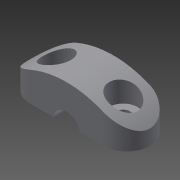
# Autodesk Inventor part: YAxisRodClamp
Saved by Autodesk Inventor 2015 (Build 190159000, 159)
## iProperties
Created: 2014-08-08
Part Number: YAxisRodClamp
Material: Generic
Document SubType Name: Modeling
Designer: t_clevj
Density: 1 g/cm^3
Appearance: Default
Author: t_clevj
Autodesk Inventor part; units mm, degrees
ref_plane "YZ Plane" through (0, 0, 0) normal (1, 0, 0) x (0, 1, 0)
ref_plane "XZ Plane" through (0, 0, 0) normal (0, 1, 0) x (-1, 0, 0)
ref_plane "XY Plane" through (0, 0, 0) normal (0, 0, 1) x (1, 0, 0)
sketch "Sketch1" plane through (0, 0, 0) normal (0, 1, 0) x (-1, 0, 0)
  line L0 (0, 0) -> (0, 4.5)
  line L1 (36, 0) -> (36, 4.5)
  arc A0 (36, 4.5) -> (0, 4.5) centre (18, -16.9476) ccw
  circle A1 centre (18, -0.6) radius 4
  line L2 (0, 0) -> (14.0453, 0)
  line L3 (36, 0) -> (21.9547, 0)
  dimension "d0" = 4.5
  dimension "d1" = 4.5
  dimension "d2" = 36
  dimension "d3" = 28
  dimension "d4" = 8
  dimension "d5" = 0.6
  dimension "d6" = 18
  constraints: 8 end point, 4 point on circle, 2 centre point, 2 vertical, 1 collinear, 1 horizontal, 1 point on line
  measures "d0" distance of L0.start L0.end
  measures "d1" distance of L1.start L1.end
  measures "d2" distance between parallel lines of L0 L1
  measures "d3" radius of A0
  measures "d4" diameter of A1
  measures "d5" vertical distance of L0.start A1.centre
  measures "d6" horizontal distance of L1.start A1.centre
extrude "Extrusion1" add sketch "Sketch1" along normal blind 14 contours L0 A0 L1 L3 A1 L2
fillet "Fillet1" radius 7 4 edges at (0, 14, 2.25) (0, 0, 2.25) (-36, 14, 2.25) (-36, 0, 2.25)
sketch "Sketch2" plane through (-14.0453, 0, 0) normal (0, 0, -1) x (-1, 0, 0)
  arc A0 (-7.0453, 14) -> (-7.0453, 0) centre (-7.0453, 7) ccw projected
  arc A1 (14.9547, 0) -> (14.9547, 14) centre (14.9547, 7) ccw projected
  line L0 (7.9095, 14) -> (14.9547, 14) projected
  line L1 (7.9095, 0) -> (7.9095, 14) projected
  line L2 (7.9095, 0) -> (14.9547, 0) projected
  circle A2 centre (-6.0453, 7) radius 2
  circle A3 centre (13.9547, 7) radius 2
  point P0 (-14.0453, 0)
  dimension "d19" = 4
  dimension "d20" = 4
  dimension "d22" = 20
  dimension "d23" = 1
  constraints: 2 centre point, 2 horizontal alignment
  measures "d19" diameter of A2
  measures "d20" diameter of A3
  measures "d22" distance of A3.centre A2.centre
  measures "d23" distance of A3.centre A1.centre
extrude "Extrusion2" cut sketch "Sketch2" against normal up to next contours A2 | A3
ref_plane "Work Plane1" through (-14.0453, 0, 4) normal (0, 0, -1) x (-1, 0, 0)
ref_plane "Work Plane2" through (-14.0453, 0, 4) normal (0, 0, -1) x (-1, 0, 0)
sketch "Sketch4" plane through (-14.0453, 0, 4) normal (0, 0, -1) x (-1, 0, 0)
  spline S0 degree 8 poles (-4.0453, 7) (-4.0453, 7.2106) (-4.0706, 7.4217) (-4.1215, 7.6308) (-4.1983, 7.8352) (-4.3013, 8.0322) (-4.4309, 8.2183) (-4.5873, 8.3896) (-4.9297, 8.6728) (-5.1107, 8.7908) (-5.3107, 8.8886) (-5.5255, 8.9613) (-5.7497, 9.0058) (-5.9775, 9.0205) (-6.2028, 9.006) (-6.6538, 8.92) (-6.8753, 8.8448) (-7.0808, 8.7428) (-7.2677, 8.6177) (-7.4339, 8.4735) (-7.5781, 8.3138) (-7.6994, 8.1426) (-7.9062, 7.7665) (-7.9875, 7.5586) (-8.0417, 7.3434) (-8.0687, 7.124) (-8.0685, 6.9033) (-8.0411, 6.6843) (-7.9865, 6.47) (-7.8339, 6.0848) (-7.7425, 5.9113) (-7.6304, 5.7458) (-7.498, 5.5912) (-7.3457, 5.4501) (-7.1746, 5.3258) (-6.9859, 5.2214) (-6.584, 5.0623) (-6.3712, 5.0057) (-6.148, 4.9757) (-5.9201, 4.9747) (-5.6938, 5.0036) (-5.4751, 5.0611) (-5.2697, 5.1441) (-4.8226, 5.3899) (-4.5988, 5.5699) (-4.4125, 5.7777) (-4.2643, 6.0055) (-4.1541, 6.2469) (-4.0813, 6.4964) (-4.0453, 6.7489) (-4.0453, 7) knots 0 0 0 0 0 0 0 0 0 0.147327 0.147327 0.147327 0.147327 0.147327 0.147327 0.147327 0.27552 0.27552 0.27552 0.27552 0.27552 0.27552 0.27552 0.413502 0.413502 0.413502 0.413502 0.413502 0.413502 0.413502 0.565351 0.565351 0.565351 0.565351 0.565351 0.565351 0.565351 0.6971 0.6971 0.6971 0.6971 0.6971 0.6971 0.6971 0.824412 0.824412 0.824412 0.824412 0.824412 0.824412 0.824412 1 1 1 1 1 1 1 1 1 projected
  circle A0 centre (-6.0453, 7) radius 2 projected
  spline S1 degree 8 poles (15.9547, 7) (15.9547, 7.1989) (15.9321, 7.3978) (15.8869, 7.5946) (15.819, 7.7868) (15.7286, 7.972) (15.6157, 8.1477) (15.4806, 8.3108) (15.1856, 8.5878) (15.0291, 8.7065) (14.8557, 8.81) (14.6674, 8.8947) (14.4671, 8.9577) (14.258, 8.9965) (14.0441, 9.0096) (13.641, 8.9842) (13.4542, 8.9521) (13.2712, 8.8999) (13.0945, 8.8282) (12.9266, 8.7378) (12.7697, 8.63) (12.6258, 8.5065) (12.3678, 8.2317) (12.2535, 8.0804) (12.1559, 7.917) (12.0762, 7.7438) (12.0157, 7.563) (11.975, 7.377) (11.9547, 7.1885) (11.9547, 6.7894) (11.9801, 6.5783) (12.031, 6.3692) (12.1077, 6.1648) (12.2108, 5.9678) (12.3404, 5.7817) (12.4968, 5.6104) (12.8392, 5.3272) (13.0202, 5.2092) (13.2202, 5.1114) (13.435, 5.0387) (13.6592, 4.9942) (13.887, 4.9795) (14.1123, 4.994) (14.7122, 5.1084) (15.0581, 5.2627) (15.3546, 5.4793) (15.5951, 5.7426) (15.7759, 6.0386) (15.8957, 6.3545) (15.9547, 6.6786) (15.9547, 7) knots 0 0 0 0 0 0 0 0 0 0.157083 0.157083 0.157083 0.157083 0.157083 0.157083 0.157083 0.295677 0.295677 0.295677 0.295677 0.295677 0.295677 0.295677 0.417006 0.417006 0.417006 0.417006 0.417006 0.417006 0.417006 0.538375 0.538375 0.538375 0.538375 0.538375 0.538375 0.538375 0.674031 0.674031 0.674031 0.674031 0.674031 0.674031 0.674031 0.792069 0.792069 0.792069 0.792069 0.792069 0.792069 0.792069 1 1 1 1 1 1 1 1 1 projected
  circle A1 centre (13.9547, 7) radius 2 projected
  circle A2 centre (-6.0453, 7) radius 4.25
  circle A3 centre (13.9547, 7) radius 4.25
  point P0 (-14.0453, 0)
  dimension "d25" = 8.5
  dimension "d26" = 8.5
  constraints: 2 centre point, 2 coincident, 2 other
  measures "d25" diameter of A2
  measures "d26" diameter of A3
extrude "Extrusion4" cut sketch "Sketch4" against normal up to next
body "Solid1"
